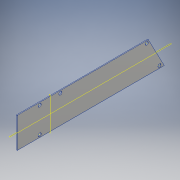
# Autodesk Inventor part: Storage Side Plate
Saved by Autodesk Inventor 2019.4 (Build 234330000, 330)
## iProperties
Created: 2020-01-24
Part Number: Storage Side Plate
Material: Aluminum 6061
Document SubType Name: Modeling
Designer: admin
Density: 2.7 g/cm^3
Appearance: Aluminum - Flat
Author: admin
Autodesk Inventor part; units mm, degrees
ref_plane "YZ Plane" through (0, 0, 0) normal (1, 0, 0) x (0, 1, 0)
ref_plane "XZ Plane" through (0, 0, 0) normal (0, 1, 0) x (-1, 0, 0)
ref_plane "XY Plane" through (0, 0, 0) normal (0, 0, 1) x (1, 0, 0)
sketch "Sketch1" plane through (0, 0, 0) normal (1, 0, 0) x (0, 1, 0)
  line L0 (0, 0) -> (190, 0)
  line L1 (190, 0) -> (190, -820)
  line L2 (190, -820) -> (0, -920)
  line L3 (0, -920) -> (0, 0)
  circle A0 centre (95, -413.3735) radius 88.9 construction
  circle A1 centre (175, -140) radius 9.5
  circle A2 centre (15, -140) radius 9.5
  circle A3 centre (15, -890) radius 9.5
  circle A4 centre (175, -810) radius 9.5
  line L4 (15, -140) -> (15, -890) construction
  line L5 (234.971, -205) -> (-89.3496, -205) construction
  circle A5 centre (175, -270) radius 9.5
  line L6 (175, -270) -> (175, -810) construction
  line L7 (15, -140) -> (175, -140) construction
  circle A6 centre (97.3586, -237.1878) radius 88.9 construction
  circle A7 centre (99.6878, -594.5711) radius 88.9 construction
  circle A8 centre (95, -787.6266) radius 88.9 construction
  dimension "d0" = 920
  dimension "d1" = 177.8
  dimension "d2" = 19
  dimension "d3" = 19
  dimension "d4" = 19
  dimension "d5" = 19
  dimension "d6" = 15
  dimension "d8" = 140
  dimension "d9" = 140
  dimension "d10" = 205
  dimension "d11" = 19
  dimension "d12" = 15
  dimension "d14" = 65
  dimension "d15" = 190
  dimension "d16" = 100
  dimension "d19" = 160
  dimension "d20" = 540
  dimension "d21" = 750
  dimension "d22" = 177.8
  dimension "d23" = 177.8
  dimension "d24" = 177.8
  constraints: 16 end point, 9 centre point, 2 horizontal, 2 vertical, 1 parallel, 1 perpendicular
  measures "d0" distance of L2.end L0.start
  measures "d1" diameter of A0
  measures "d2" diameter of A1
  measures "d3" diameter of A2
  measures "d4" diameter of A3
  measures "d5" diameter of A4
  measures "d6" distance between parallel lines of L3 L4
  measures "d8" distance from line of L0 L7.end
  measures "d9" distance from line of L0 L4.start
  measures "d10" distance between parallel lines of L0 L5
  measures "d11" diameter of A5
  measures "d12" distance between parallel lines of L1 L6
  measures "d14" distance from line of L5 L6.start
  measures "d15" distance of L0.start L0.end
  measures "d16" vertical distance of L1.end L2.end
  measures "d19" distance of L4.start L7.end
  measures "d20" distance of L6.start L6.end
  measures "d21" distance of L4.start L4.end
  measures "d22" diameter of A6
  measures "d23" diameter of A7
  measures "d24" diameter of A8
extrude "Extrusion1" add sketch "Sketch1" along normal blind 5
ref_plane "Work Plane3" through (5, 95, -140) normal (0, -1, 0) x (-1, 0, 0)
ref_plane "Work Plane1" through (5, 175, -140) normal (0, -1, 0) x (-1, 0, 0)
ref_plane "Work Plane2" through (5, 15, -890) normal (0, 1, 0) x (-1, 0, 0)
ref_plane "Work Plane5" through (5, 175, -205) normal (0, 0, 1) x (-1, 0, 0)
ref_plane "Work Plane4" through (5, 175, -140) normal (0, 0, 1) x (-1, 0, 0)
body "Solid1"
